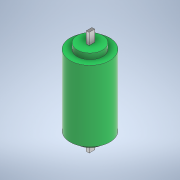
# Autodesk Inventor part: tilt
Saved by Autodesk Inventor 2021 (Build 250183000, 183)
## iProperties
Created: 2021-07-15
Part Number: tilt
Material: Generic
Document SubType Name: Modeling
Designer: HP
Density: 1 g/cm^3
Appearance: Default
Author: HP
Autodesk Inventor part; units mm, degrees
ref_plane "YZ Plane" through (0, 0, 0) normal (1, 0, 0) x (0, 1, 0)
ref_plane "XZ Plane" through (0, 0, 0) normal (0, 1, 0) x (-1, 0, 0)
ref_plane "XY Plane" through (0, 0, 0) normal (0, 0, 1) x (1, 0, 0)
sketch "Sketch1" plane through (0, 0, 0) normal (0, 1, 0) x (-1, 0, 0)
  circle A0 centre (0, 0) radius 7
  dimension "d0" = 14
  constraints: 1 centre point, 1 coincident
  measures "d0" diameter of A0
extrude "Extrusion1" add sketch "Sketch1" along normal blind 25
sketch "Sketch2" plane through (0, 25, 0) normal (0, 1, 0) x (1, 0, 0)
  circle A0 centre (0, 0) radius 4.5
  dimension "d3" = 9
  constraints: 1 centre point, 1 coincident
  measures "d3" diameter of A0
sketch "Sketch3" plane through (0, 0, 0) normal (0, -1, 0) x (1, 0, 0)
  circle A0 centre (0, 0) radius 4.5
  dimension "d4" = 9
  constraints: 1 centre point, 1 coincident
  measures "d4" diameter of A0
extrude "Extrusion2" add sketch "Sketch3" along normal mid plane 4
extrude "Extrusion3" add sketch "Sketch2" along normal blind 2
sketch "Sketch4" plane through (0, -2, 0) normal (0, -1, 0) x (1, 0, 0)
  line L0 (-0.3275, -1.0042) -> (0.6725, -1.0042)
  line L1 (0.6725, -1.0042) -> (0.6725, 0.9958)
  line L2 (0.6725, 0.9958) -> (-0.3275, 0.9958)
  line L3 (-0.3275, 0.9958) -> (-0.3275, -1.0042)
  point P0 (0, 0)
  dimension "d9" = 1
  dimension "d10" = 2
  constraints: 8 end point, 2 parallel, 1 horizontal, 1 perpendicular
  measures "d9" distance of L2.end L1.end
  measures "d10" distance of L1.end L0.end
extrude "Extrusion4" add sketch "Sketch4" along normal blind 4
sketch "Sketch5" plane through (0, 27, 0) normal (0, 1, 0) x (1, 0, 0)
  line L0 (0.6725, -0.9958) -> (-0.3275, -0.9958) projected
  line L1 (0.6725, 1.0042) -> (0.6725, -0.9958) projected
  line L2 (-0.3275, -0.9958) -> (0.6725, -0.9958)
  line L3 (0.6725, -0.9958) -> (0.6725, 1.0042)
  line L4 (0.6725, 1.0042) -> (-0.3275, 1.0042)
  line L5 (-0.3275, 1.0042) -> (-0.3275, -0.9958)
  point P0 (0, 0)
  constraints: 8 end point, 2 parallel, 1 horizontal, 1 perpendicular
extrude "Extrusion5" add sketch "Sketch5" along normal blind 4
body "Solid1"
